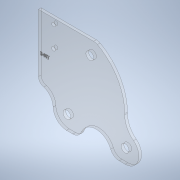
# Autodesk Inventor part: Intake Sides V6ipt
Saved by Autodesk Inventor 2022 (Build 260153000, 153)
## iProperties
Created: 2022-10-16
Part Number: Intake Sides V6ipt
Material: Polycarbonate, Clear
Document SubType Name: Modeling
Designer: matt
Density: 1.2 g/cm^3
Appearance: Polycarbonate - Clear
Mass: 60.255 g
Surface Area: 348.282 cm^2
Volume: 50.2125 cm^3
Author: matt
Autodesk Inventor part; units mm, degrees
ref_plane "YZ Plane" through (0, 0, 0) normal (1, 0, 0) x (0, 1, 0)
ref_plane "XZ Plane" through (0, 0, 0) normal (0, 1, 0) x (-1, 0, 0)
ref_plane "XY Plane" through (0, 0, 0) normal (0, 0, 1) x (1, 0, 0)
sketch "Sketch1" plane through (0, 0, 0) normal (0, 0, 1) x (1, 0, 0)
  line L0 (131.3749, -73.5016) -> (131.3749, -71.6344)
  arc A0 (131.3749, -71.6344) -> (89.8052, -1.2952) centre (51.0805, -71.6344) ccw
  arc A1 (89.8052, -1.2952) -> (84.0169, -0.1805) centre (84.7113, -12.1604) ccw
  line L1 (84.0169, -0.1805) -> (0.0993, 0.1926)
  line L2 (0.0993, 0.1926) -> (-0.2975, -89.0508)
  arc A2 (-0.2975, -89.0508) -> (7.9081, -98.4818) centre (9.6942, -88.6426) ccw
  circle A3 centre (120.9184, -82.9714) radius 3.3
  arc A4 (145.7873, -114.287) -> (148.0883, -110.4202) centre (146.9636, -112.3689) ccw
  arc A5 (145.7873, -124.287) -> (148.0882, -120.4202) centre (146.9636, -122.3689) ccw
  circle A6 centre (22.531, -40.6102) radius 2.8
  circle A7 centre (28.6758, -122.3689) radius 2.25
  circle A8 centre (28.6758, -112.3689) radius 2.25
  circle A9 centre (10, -88.6441) radius 3.3
  arc A10 (32.2446, -127.2916) -> (33.2446, -128.2916) centre (33.2446, -127.2916) ccw
  line L3 (32.2446, -127.2916) -> (32.2446, -107.4916)
  arc A11 (33.2446, -106.4916) -> (32.2446, -107.4916) centre (33.2446, -107.4916) ccw
  arc A12 (142.8483, -107.4916) -> (141.8483, -106.4916) centre (141.8483, -107.4916) ccw
  line L4 (142.8483, -107.4916) -> (142.8483, -127.2916)
  arc A13 (141.8483, -128.2916) -> (142.8483, -127.2916) centre (141.8483, -127.2916) ccw
  circle A14 centre (146.9636, -112.3689) radius 2.25
  circle A15 centre (146.9636, -122.3689) radius 2.25
  circle A16 centre (43.0964, -117.3689) radius 6
  circle A17 centre (131.9964, -117.3688) radius 6
  circle A18 centre (78.1699, -22.3386) radius 3.25
  circle A19 centre (78.1699, -22.3386) radius 6
  arc A20 (131.9964, -138.3688) -> (144.7874, -100.7138) centre (131.9964, -117.3688) ccw
  arc A21 (22.0858, -117.7084) -> (7.9081, -98.4818) centre (1.5094, -118.0409) ccw
  arc A22 (131.3749, -73.5016) -> (144.7874, -100.7138) centre (165.6862, -73.5016) ccw
  arc A23 (22.0858, -117.7084) -> (42.3476, -138.3689) centre (43.0964, -117.3689) ccw
  arc A24 (109.9151, -129.4423) -> (65.1778, -129.4423) centre (87.5464, -138.1396) ccw
  line L5 (42.3476, -138.3689) -> (52.1294, -138.3689)
  line L6 (122.9635, -138.3688) -> (131.9964, -138.3688)
  arc A25 (52.1294, -138.3689) -> (65.1778, -129.4423) centre (52.1294, -124.3689) ccw
  arc A26 (109.9151, -129.4423) -> (122.9635, -138.3688) centre (122.9635, -124.3688) ccw
  circle A27 centre (43.0964, -117.3689) radius 4.6 projected
  line L7 (1.9461, -54.0938) -> (33.2975, -54.0938) construction
  line L8 (33.2975, -54.0938) -> (33.2975, -61.1615) construction
  line L9 (33.2975, -61.1615) -> (1.9461, -61.1615) construction
  line L10 (1.9461, -61.1615) -> (1.9461, -54.0938) construction
  circle A28 centre (79.294, -41.6199) radius 2.8
  circle A29 centre (78.1699, -22.3386) radius 6
  circle A30 centre (22.531, -40.6102) radius 2.8
  circle A31 centre (22.6705, -8.6105) radius 2.8
  circle A32 centre (22.6705, -8.6105) radius 2.8
  circle A33 centre (120.9184, -82.9714) radius 3.3
  line L11 (2.1801, -54.1888) -> (3.0075, -54.1888)
  spline S0 degree 2 poles (3.0075, -54.1888) (3.8349, -54.1888) (4.4216, -54.3176) (4.7912, -54.8433) (4.7912, -55.4164) knots 0 0 0 1 2 3 3 3
  spline S1 degree 2 poles (4.7912, -55.4164) (4.7912, -55.942) (4.5301, -56.3048) (4.1469, -56.3421) knots 0 0 0 1 2 2 2
  spline S2 degree 2 poles (4.1469, -56.3421) (4.4928, -56.4269) (4.7336, -56.7152) (4.7912, -56.9559) (4.7912, -57.5019) knots 0 0 0 1 2 3 3 3
  line L12 (4.7912, -57.5019) -> (4.7912, -58.6888)
  line L13 (4.7912, -58.6888) -> (3.7027, -58.6888)
  line L14 (3.7027, -58.6888) -> (3.7027, -57.1933)
  spline S3 degree 2 poles (3.7027, -57.1933) (3.7027, -56.8338) (3.5908, -56.6609) (3.35, -56.6609) knots 0 0 0 1 2 2 2
  line L15 (3.35, -56.6609) -> (3.35, -58.6888)
  line L16 (3.35, -58.6888) -> (2.1801, -58.6888)
  line L17 (2.1801, -58.6888) -> (2.1801, -54.1888)
  line L18 (3.35, -54.9586) -> (3.35, -55.9589)
  spline S4 degree 2 poles (3.35, -55.9589) (3.5467, -55.9589) (3.7027, -55.8504) (3.7027, -55.552) knots 0 0 0 1 2 2 2
  line L19 (3.7027, -55.552) -> (3.7027, -55.3045)
  spline S5 degree 2 poles (3.7027, -55.3045) (3.7027, -55.0908) (3.5501, -54.9586) (3.35, -54.9586) knots 0 0 0 1 2 2 2
  line L20 (6.5851, -56.454) -> (6.5851, -57.2306)
  line L21 (6.5851, -57.2306) -> (5.1134, -57.2306)
  line L22 (5.1134, -57.2306) -> (5.1134, -56.454)
  line L23 (5.1134, -56.454) -> (6.5851, -56.454)
  spline S6 degree 2 poles (9.593, -56.8237) (9.593, -57.5019) (9.5286, -58.0648) (9.1929, -58.5328) (8.6198, -58.7837) (8.24, -58.7837) knots 0 0 0 1 2 3 4 4 4
  spline S7 degree 2 poles (8.24, -58.7837) (7.8771, -58.7837) (7.304, -58.5464) (6.9548, -58.075) (6.8869, -57.5189) (6.8869, -56.8237) knots 0 0 0 1 2 3 4 4 4
  line L24 (6.8869, -56.8237) -> (6.8869, -56.0539)
  spline S8 degree 2 poles (6.8869, -56.0539) (6.8869, -55.3757) (6.9514, -54.8127) (7.2871, -54.3448) (7.8602, -54.0938) (8.24, -54.0938) knots 0 0 0 1 2 3 4 4 4
  spline S9 degree 2 poles (8.24, -54.0938) (8.6028, -54.0938) (9.1759, -54.3312) (9.5252, -54.8026) (9.593, -55.3587) (9.593, -56.0539) knots 0 0 0 1 2 3 4 4 4
  line L25 (9.593, -56.0539) -> (9.593, -56.8237)
  spline S10 degree 2 poles (8.4231, -55.3452) (8.4231, -55.0332) (8.3553, -54.8568) (8.2468, -54.8568) knots 0 0 0 1 2 2 2
  spline S11 degree 2 poles (8.2468, -54.8568) (8.1552, -54.8568) (8.0569, -54.9993) (8.0569, -55.3452) knots 0 0 0 1 2 2 2
  line L26 (8.0569, -55.3452) -> (8.0569, -57.4442)
  spline S12 degree 2 poles (8.0569, -57.4442) (8.0569, -57.8376) (8.1213, -58.0207) (8.2366, -58.0207) knots 0 0 0 1 2 2 2
  spline S13 degree 2 poles (8.2366, -58.0207) (8.3553, -58.0207) (8.4231, -57.8105) (8.4231, -57.4137) knots 0 0 0 1 2 2 2
  line L27 (8.4231, -57.4137) -> (8.4231, -55.3452)
  line L28 (12.6891, -54.1888) -> (12.6891, -57.1967)
  spline S14 degree 2 poles (12.6891, -57.1967) (12.6891, -57.7088) (12.6213, -58.1225) (12.2958, -58.5599) (11.76, -58.7837) (11.3937, -58.7837) knots 0 0 0 1 2 3 4 4 4
  spline S15 degree 2 poles (11.3937, -58.7837) (10.9902, -58.7837) (10.3764, -58.5158) (10.0678, -58.0886) (10.0135, -57.6138) (10.0135, -56.8508) knots 0 0 0 1 2 3 4 4 4
  line L29 (10.0135, -56.8508) -> (10.0135, -54.1888)
  line L30 (10.0135, -54.1888) -> (11.1835, -54.1888)
  line L31 (11.1835, -54.1888) -> (11.1835, -57.5629)
  spline S16 degree 2 poles (11.1835, -57.5629) (11.1835, -57.858) (11.2479, -58.0207) (11.3429, -58.0207) knots 0 0 0 1 2 2 2
  spline S17 degree 2 poles (11.3429, -58.0207) (11.4548, -58.0207) (11.5192, -57.841) (11.5192, -57.5053) knots 0 0 0 1 2 2 2
  line L32 (11.5192, -57.5053) -> (11.5192, -54.1888)
  line L33 (11.5192, -54.1888) -> (12.6891, -54.1888)
  line L34 (15.5004, -54.1888) -> (15.5004, -55.0908)
  line L35 (15.5004, -55.0908) -> (14.8052, -55.0908)
  line L36 (14.8052, -55.0908) -> (14.8052, -58.6888)
  line L37 (14.8052, -58.6888) -> (13.6352, -58.6888)
  line L38 (13.6352, -58.6888) -> (13.6352, -55.0908)
  line L39 (13.6352, -55.0908) -> (12.9435, -55.0908)
  line L40 (12.9435, -55.0908) -> (12.9435, -54.1888)
  line L41 (12.9435, -54.1888) -> (15.5004, -54.1888)
  point P0 (0, 0)
  point P1 (58.8546, -117.3689)
  point P2 (63.5475, -138.3689)
  point P3 (111.5453, -138.3689)
  dimension "d6" = 10
  dimension "d7" = 12
  dimension "d10" = 88.9
  dimension "d11" = 42
  dimension "d13" = 10.8518
  dimension "d14" = 10.8518
  dimension "d16" = 4.1153
  dimension "d17" = 4.1153
  dimension "d18" = 48
  dimension "d19" = 14
  dimension "d20" = 44.45
  dimension "d23" = 5.6
  dimension "d25" = 56.763
  dimension "d26" = 19.314
  dimension "d27" = 78.17
  constraints: 34 point on circle, 33 centre point, 14 end point, 9 coincident, 8 tangent, 3 equal radius, 2 point on line, 1 perpendicular, 12 other
  measures "d6" distance of A7.centre A8.centre
  measures "d7" diameter of A19
  measures "d10" distance of A17.centre A16.centre
  measures "d11" diameter of A20
  measures "d13" distance from line of L3 A16.centre
  measures "d14" distance from line of L4 A17.centre
  measures "d16" distance from line of L4 A14.centre
  measures "d17" distance from line of L4 A15.centre
  measures "d18" diameter of A24
  measures "d19" radius of A25
  measures "d20" horizontal distance of A24.centre A16.centre
  measures "d23" diameter of A28
  measures "d25" horizontal distance of A28.centre A6.centre
  measures "d26" distance of A28.centre A19.centre
  measures "d27" distance from line of L2 A19.centre
extrude "Extrusion1" add sketch "Sketch1" along normal blind 4.1153 contours A22 A20 L6 A26 A24 A25 L5 A23 A21 A2 L2 L1 A1 A0 L0 | A14 A4 | A15 A5 | A7 | A8 | A9 | L11 S0 S1 S2 L12 L13 L14 S3 L15 L16 L17 | S5 L19 S4 L18 | L20 L21 L22 L23 | S6 S7 L24 S8 S9 L25 | L27 S13 S12 L26 S11 S10 | L28 S14 S15 L29 L30 L31 S16 S17 L32 L33 | L34 L35 L36 L37 L38 L39 L40 L41
extrude "Extrusion2" cut sketch "Sketch1" against normal blind 1 from surface at 4.1153 contours L11 S0 S1 S2 L12 L13 L14 S3 L15 L16 L17 | L20 L21 L22 L23 | S6 S7 L24 S8 S9 L25 | L28 S14 S15 L29 L30 L31 S16 S17 L32 L33 | L34 L35 L36 L37 L38 L39 L40 L41
equation "\"d14\" = d13"
equation "\"d16\" = d15"
equation "\"d17\" = d15"
equation "\"d20\" = 0.5 * d10"
equation "\"d0\" = d16"
equation "\"d15\" = 4.115311"
body "Solid1"
